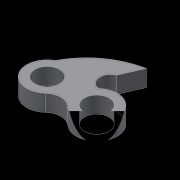
# Autodesk Inventor part: ChainTooth
Saved by Autodesk Inventor 2015 (Build 190159000, 159)
## iProperties
Created: 2015-07-29
Part Number: ChainTooth
Material: Generic
Document SubType Name: Modeling
Designer: Val
Density: 1 g/cm^3
Appearance: Default
Author: Val
Autodesk Inventor part; units mm, degrees
ref_plane "YZ Plane" through (0, 0, 0) normal (1, 0, 0) x (0, 1, 0)
ref_plane "XZ Plane" through (0, 0, 0) normal (0, 1, 0) x (-1, 0, 0)
ref_plane "XY Plane" through (0, 0, 0) normal (0, 0, 1) x (1, 0, 0)
sketch "Body" plane through (0, 0, 0) normal (0, 0, 1) x (1, 0, 0)
  circle A0 centre (0, 0) radius 0.75
  line L0 (0, 0) -> (3, 0) construction
  circle A1 centre (3, 0) radius 0.75
  arc A2 (0.8721, 0.8955) -> (0.8721, -0.8955) centre (0, 0) ccw
  arc A3 (2.1279, -0.8955) -> (2.1279, 0.8955) centre (3, 0) ccw
  arc A4 (0.8721, 0.8955) -> (2.1279, 0.8955) centre (1.5, 1.5403) ccw
  arc A5 (2.1279, -0.8955) -> (0.8721, -0.8955) centre (1.5, -1.5403) ccw
  arc A6 (2.5811, 3.4282) -> (-0.6, 1.0966) centre (3.3817, -1) ccw
  line L1 (2.5811, 3.4282) -> (2.0129, 2.1216)
  arc A7 (2.0129, 2.1216) -> (2.1279, 0.8955) centre (2.2472, 1.5251) ccw
  dimension "d0" = 1.5
  dimension "d1" = 3
  dimension "d3" = 2.5
  dimension "d5" = 0.9
  dimension "d8" = 4.5
  dimension "d10" = 113.5
  dimension "d13" = 1
  dimension "d15" = 0.6408
  dimension "d16" = 1
  dimension "d17" = 2.5
  dimension "d18" = 0.4526
  constraints: 13 point on circle, 8 centre point, 4 coincident, 4 end point, 3 symmetric about line, 2 equal radius, 2 tangent, 1 horizontal, 1 other
  measures "d0" diameter of A0
  measures "d1" distance of L0.start L0.end
  measures "d3" diameter of A2
  measures "d5" radius of A4
  measures "d8" radius of A6
  measures "d10" angle of L1 L0
  measures "d13" distance from line of A6.centre L0
  measures "d15" radius of A7
  measures "d16" distance from line of point (0, 0) L1
  measures "d17" distance from line of A6.centre L1
  measures "d18" distance from line of A7.centre L1
extrude "BodyFeature" add sketch "Body" along normal blind 1
